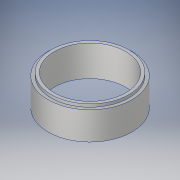
# Autodesk Inventor part: Retainer Master Sketch
Saved by Autodesk Inventor 2017 (Build 210142000, 142)
## iProperties
Created: 2016-07-25
Part Number: Retainer Master Sketch
Material: Aluminum 6061
Document SubType Name: Modeling
Designer: Jared
Density: 2.7 g/cm^3
Appearance: Aluminum - Flat
Author: Jared
Autodesk Inventor part; units mm, degrees
ref_plane "YZ Plane" through (0, 0, 0) normal (1, 0, 0) x (0, 1, 0)
ref_plane "XZ Plane" through (0, 0, 0) normal (0, 1, 0) x (-1, 0, 0)
ref_plane "XY Plane" through (0, 0, 0) normal (0, 0, 1) x (1, 0, 0)
sketch "Sketch1" plane through (0, 0, 0) normal (0, 0, 1) x (1, 0, 0)
  line L0 (0, 25.4) -> (-28.702, 25.4) construction
  line L1 (0, 25.4) -> (-86.36, 25.4) construction
  line L2 (-86.36, 25.4) -> (-80.01, 25.4) construction
  line L3 (-80.01, 25.4) -> (-73.66, 22.4389) construction
  line L4 (-80.01, 25.4) -> (-80.01, 22.4389) construction
  line L5 (-80.01, 0) -> (-86.36, 0)
  line L6 (-28.702, 59.6457) -> (-28.702, -91.9304) construction
  arc A0 (-28.9184, -4.2142) -> (-32.3684, 3.1843) centre (-35.052, -2.5707) ccw
  line L7 (-67.31, -147.4937) -> (-28.9184, -4.2142)
  line L8 (-80.01, 22.4389) -> (-73.66, 22.4389)
  line L9 (-80.01, 22.4389) -> (-80.01, 0)
  line L10 (-73.66, 22.4389) -> (-32.3684, 3.1843)
  line L11 (-28.702, -2.5707) -> (-60.452, -2.5707) construction
  line L12 (-60.452, 16.28) -> (-60.452, -121.8993) construction
  line L13 (-60.452, -121.8993) -> (-54.102, -121.8993) construction
  line L14 (-54.102, -121.8993) -> (-54.102, -98.2008) construction
  line L15 (-54.102, -98.2008) -> (-60.452, -98.2008)
  line L16 (-60.452, 16.28) -> (-60.452, 6.755) construction
  line L17 (-60.452, 16.28) -> (-60.452, 9.93) construction
  line L18 (-60.452, 9.93) -> (-46.8344, 9.93)
  line L19 (-60.452, 9.93) -> (-60.452, -98.2008)
  line L20 (-86.36, 0) -> (-86.36, -12.7) construction
  line L21 (-60.452, -12.7) -> (-73.152, -12.7) construction
  line L22 (-86.36, -12.7) -> (-86.36, -25.4) construction
  line L23 (-86.36, -25.4) -> (-86.36, -88.9) construction
  line L24 (-86.36, -88.9) -> (-73.66, -88.9) construction
  line L25 (-73.66, -88.9) -> (-73.66, -25.4) construction
  line L26 (-86.36, -25.4) -> (-73.66, -25.4)
  line L27 (-73.66, -25.4) -> (-73.66, -88.9)
  line L28 (-73.66, -88.9) -> (-86.36, -88.9)
  line L29 (-86.36, -12.7) -> (-73.152, -12.7)
  line L30 (-73.152, -133.7486) -> (-63.627, -133.7486)
  line L31 (-73.66, -88.9) -> (-73.66, -147.4937)
  line L32 (-73.66, -147.4937) -> (-67.31, -147.4937)
  line L33 (-73.152, -12.7) -> (-73.152, -133.7486)
  line L34 (-80.01, -25.4) -> (-80.01, -31.3436)
  line L35 (-80.01, -31.3436) -> (-86.36, -31.3436)
  line L36 (-86.36, 0) -> (-86.36, -25.4)
  line L37 (-86.36, -31.3436) -> (-86.36, -88.9)
  line L38 (0, -319.0244) -> (0, 122.7573) projected
  point P0 (0, 0)
  point P1 (-86.36, -255.9127)
  point P2 (-76.835, 22.4389)
  dimension "d0" = 28.702
  dimension "d1" = 86.36
  dimension "d2" = 6.35
  dimension "d3" = 25
  dimension "d5" = 25.4
  dimension "d6" = 25.4
  dimension "d8" = 12.7
  dimension "d11" = 6.35
  dimension "d12" = 31.75
  dimension "d13" = 6.35
  dimension "d15" = 6.35
  dimension "d16" = 12.7
  dimension "d17" = 12.7
  dimension "d18" = 12.7
  dimension "d19" = 63.5
  dimension "d20" = 12.7
  dimension "d22" = 9.525
  dimension "d23" = 6.35
  dimension "d25" = 5.9436
  dimension "d26" = 15
  constraints: 76 end point, 15 perpendicular, 14 point on line, 11 vertical, 5 horizontal, 5 vertical alignment, 4 tangent, 3 midpoint, 3 point on circle, 2 collinear, 1 centre point
  measures "d0" distance of L0.start L0.end
  measures "d1" distance of L0.start L1.end
  measures "d2" distance of L1.end L2.end
  measures "d3" angle of L1 L3
  measures "d5" distance of point (0, 0) L0.start
  measures "d6" distance of L2.end L5.start
  measures "d8" diameter of A0
  measures "d11" distance of L4.end L3.end
  measures "d12" distance of L11.start L11.end
  measures "d13" distance of L12.end L13.end
  measures "d15" distance of L12.start L17.end
  measures "d16" distance of L5.end L20.end
  measures "d17" distance of L21.start L21.end
  measures "d18" distance of L20.end L22.end
  measures "d19" distance of L23.end L22.end
  measures "d20" distance of L23.end L24.end
  measures "d22" distance of L30.start L30.end
  measures "d23" distance of L31.end L7.start
  measures "d25" distance of L34.start L34.end
  measures "d26" angle of L7 L19
revolve "Revolution4" add sketch "Sketch1" angle 360 about axis through (0, -10, 0) along (0, 1, 0) contours L26 L27 L28 L37 L35 L34
body "Solid4"
